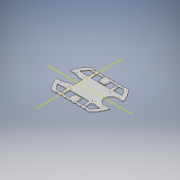
# Autodesk Inventor part: bottomPlate
Saved by Autodesk Inventor 2018 (Build 220112000, 112)
## iProperties
Created: 2020-01-08
Part Number: bottomPlate
Material: Generic
Document SubType Name: Modeling
Designer: anirudh
Density: 1 g/cm^3
Appearance: Default
Author: anirudh
Autodesk Inventor part; units mm, degrees
ref_plane "YZ Plane" through (0, 0, 0) normal (1, 0, 0) x (0, 1, 0)
ref_plane "XZ Plane" through (0, 0, 0) normal (0, 1, 0) x (-1, 0, 0)
ref_plane "XY Plane" through (0, 0, 0) normal (0, 0, 1) x (1, 0, 0)
sketch "Sketch1" plane through (0, 0, 0) normal (0, 1, 0) x (-1, 0, 0)
  arc A0 (-134.4042, 152.4) -> (-189.4285, 73.533) centre (0, 0) ccw
  arc A1 (-189.4285, -73.533) -> (-134.4042, -152.4) centre (0, 0) ccw
  arc A2 (-134.4042, 152.4) -> (-189.4285, 73.533) centre (0, 0) ccw
  arc A3 (-189.4285, -73.533) -> (-134.4042, -152.4) centre (0, 0) ccw
  arc A4 (214.8285, 73.533) -> (159.8042, 152.4) centre (25.4, 0) ccw
  arc A5 (159.8042, -152.4) -> (214.8285, -73.533) centre (25.4, 0) ccw
  arc A6 (214.8285, 73.533) -> (159.8042, 152.4) centre (25.4, 0) ccw
  arc A7 (159.8042, -152.4) -> (214.8285, -73.533) centre (25.4, 0) ccw
  arc A8 (-152.4, -50.8) -> (-152.4, 50.8) centre (-152.4, 0) ccw
  arc A9 (177.8, 50.8) -> (177.8, -50.8) centre (177.8, 0) ccw
  line L0 (177.8, 50.8) -> (222.1476, 50.8)
  line L1 (177.8, -50.8) -> (222.1476, -50.8)
  line L2 (-152.4, 50.8) -> (-196.7476, 50.8)
  line L3 (-152.4, -50.8) -> (-196.7476, -50.8)
  arc A10 (-134.4042, 152.4) -> (-196.7476, 50.8) centre (0, 0) ccw
  arc A11 (-196.7476, -50.8) -> (-134.4042, -152.4) centre (0, 0) ccw
  arc A12 (159.8042, -152.4) -> (222.1476, -50.8) centre (25.4, 0) ccw
  arc A13 (222.1476, 50.8) -> (159.8042, 152.4) centre (25.4, 0) ccw
  circle A14 centre (98.425, -65.0875) radius 2.1
  circle A15 centre (98.425, 65.0875) radius 2.1
  circle A16 centre (-73.025, 65.0875) radius 2.1
  circle A17 centre (-73.025, -65.0875) radius 2.1
  line L4 (-20.32, 152.4) -> (-20.32, 147.32)
  line L5 (-20.32, 147.32) -> (-30.48, 147.32)
  line L6 (-30.48, 147.32) -> (-30.48, 152.4)
  line L7 (-92.5481, 152.4) -> (-92.5481, 147.32)
  line L8 (-92.5481, 147.32) -> (-102.7081, 147.32)
  line L9 (-102.7081, 147.32) -> (-102.7081, 152.4)
  line L10 (-102.7081, 152.4) -> (-134.4042, 152.4)
  line L11 (-60.8521, 152.4) -> (-92.5481, 152.4)
  line L12 (-102.7081, 152.4) -> (-134.4042, 152.4)
  line L13 (-134.4042, 152.4) -> (-102.7081, 152.4)
  line L14 (12.7, 152.4) -> (-20.32, 152.4)
  line L15 (-30.48, 152.4) -> (-60.8521, 152.4)
  line L16 (12.7, 152.4) -> (-20.32, 152.4)
  line L17 (-30.48, 152.4) -> (-92.5481, 152.4)
  line L18 (-92.5481, 152.4) -> (-30.48, 152.4)
  line L19 (-20.32, 152.4) -> (12.7, 152.4)
  line L20 (45.72, 152.4) -> (45.72, 147.32)
  line L21 (45.72, 147.32) -> (55.88, 147.32)
  line L22 (55.88, 147.32) -> (55.88, 152.4)
  line L23 (117.9481, 152.4) -> (117.9481, 147.32)
  line L24 (117.9481, 147.32) -> (128.1081, 147.32)
  line L25 (128.1081, 147.32) -> (128.1081, 152.4)
  line L26 (-20.32, -152.4) -> (-20.32, -147.32)
  line L27 (-20.32, -147.32) -> (-30.48, -147.32)
  line L28 (-30.48, -147.32) -> (-30.48, -152.4)
  line L29 (-92.5481, -152.4) -> (-92.5481, -147.32)
  line L30 (-92.5481, -147.32) -> (-102.7081, -147.32)
  line L31 (-102.7081, -147.32) -> (-102.7081, -152.4)
  line L32 (55.88, -147.32) -> (55.88, -152.4)
  line L33 (45.72, -147.32) -> (55.88, -147.32)
  line L34 (45.72, -152.4) -> (45.72, -147.32)
  line L35 (117.9481, -147.32) -> (128.1081, -147.32)
  line L36 (128.1081, -147.32) -> (128.1081, -152.4)
  line L37 (117.9481, -152.4) -> (117.9481, -147.32)
  line L38 (128.1081, 152.4) -> (159.8042, 152.4)
  line L39 (12.7, 152.4) -> (45.72, 152.4)
  line L40 (55.88, 152.4) -> (117.9481, 152.4)
  line L41 (-102.7081, -152.4) -> (-134.4042, -152.4)
  line L42 (12.7, -152.4) -> (-20.32, -152.4)
  line L43 (-30.48, -152.4) -> (-92.5481, -152.4)
  line L44 (12.7, -152.4) -> (45.72, -152.4)
  line L45 (55.88, -152.4) -> (117.9481, -152.4)
  line L46 (128.1081, -152.4) -> (159.8042, -152.4)
  point P0 (-25.4, -152.4)
  point P1 (50.8, 152.4)
  point P2 (50.8, -152.4)
  point P3 (50.8, -152.4)
  dimension "d22" = 101.6
  dimension "d31" = 4.2
  dimension "d32" = 4.2
  dimension "d34" = 4.2
  constraints: 94 end point, 28 point on circle, 18 centre point, 15 collinear, 12 point on line, 7 perpendicular, 4 coincident, 2 tangent, 1 vertical
  measures "d22" diameter of A9
  measures "d31" diameter of A14
  measures "d32" diameter of A15
  measures "d34" diameter of A17
extrude "Extrusion2" add sketch "Sketch1" along normal blind 5.08
sketch "Sketch2" plane through (0, 5.08, 0) normal (0, 1, 0) x (1, 0, 0)
  arc A0 (-177.8, -50.8) -> (-177.8, 50.8) centre (-177.8, 0) ccw projected
  arc A1 (152.4, 50.8) -> (152.4, -50.8) centre (152.4, 0) ccw projected
  line L0 (-177.8, 0) -> (152.4, 0)
  line L1 (-12.7, 0) -> (-12.7, -152.4)
  line L2 (-12.7, 0) -> (-12.7, 152.4)
  line L3 (20.32, 152.4) -> (-45.72, 152.4) projected
  point P0 (0, 0)
  constraints: 6 end point, 2 midpoint, 1 horizontal
sketch "Sketch3" plane through (0, 5.08, 0) normal (0, 1, 0) x (1, 0, 0)
  circle A0 centre (9.525, 140.4366) radius 1.75
  circle A1 centre (-34.925, 140.4366) radius 1.75
  circle A2 centre (9.525, 102.362) radius 1.75
  circle A3 centre (-34.925, 102.362) radius 1.75
  arc A4 (152.4, 50.8) -> (152.4, -50.8) centre (152.4, 0) ccw projected
  circle A5 centre (9.525, -140.4366) radius 1.75
  circle A6 centre (-34.925, -140.4366) radius 1.75
  circle A7 centre (9.525, -102.362) radius 1.75
  circle A8 centre (-34.925, -102.362) radius 1.75
  point P0 (0, 0)
  dimension "d56" = 3.5
  dimension "d57" = 3.5
  dimension "d58" = 3.5
  constraints: 8 centre point
  measures "d56" diameter of A1
  measures "d57" diameter of A2
  measures "d58" diameter of A3
extrude "Extrusion3" cut sketch "Sketch3" against normal blind 25.4
sketch "Sketch4" plane through (0, 5.08, 0) normal (0, 1, 0) x (1, 0, 0)
  circle A0 centre (-12.7, 0) radius 300
  point P0 (-177.8, 0)
  point P1 (152.4, 0)
  constraints: 1 centre point
sketch "Sketch5" plane through (0, 5.08, 0) normal (0, 1, 0) x (1, 0, 0)
  line L0 (101.6, 0) -> (80.9498, 0)
  arc A0 (-177.8, -50.8) -> (-177.8, 50.8) centre (-177.8, 0) ccw projected
  line L1 (-106.3498, 0) -> (-106.3498, -74.5998)
  line L2 (30.48, -152.4) -> (92.5481, -152.4) projected
  line L3 (80.9498, -74.5998) -> (-106.3498, -74.5998)
  line L4 (-55.88, 152.4) -> (-117.9481, 152.4) projected
  line L5 (-106.3498, 74.5998) -> (80.9498, 74.5998)
  circle A1 centre (9.525, -102.362) radius 1.75 projected
  line L6 (20.32, 152.4) -> (-45.72, 152.4) projected
  circle A2 centre (-34.925, -140.4366) radius 1.75 projected
  line L7 (-41.3004, -140.4366) -> (-41.3004, -152.4)
  line L8 (-45.72, -152.4) -> (20.32, -152.4) projected
  circle A3 centre (-34.925, -102.362) radius 1.75 projected
  line L9 (-34.925, -89.6366) -> (-41.3004, -89.6366)
  line L10 (-41.3004, -89.6366) -> (15.9004, -89.6366)
  circle A4 centre (-34.925, 102.362) radius 1.75 projected
  line L11 (-34.925, 89.6366) -> (-41.3004, 89.6366)
  line L12 (-41.3004, 89.6366) -> (15.9004, 89.6366)
  line L13 (-41.3004, -152.4) -> (-41.3004, -89.6366)
  line L14 (-41.3004, 89.6366) -> (-41.3004, 152.4)
  line L15 (15.9004, -152.4) -> (15.9004, -89.6366)
  line L16 (15.9004, 89.6366) -> (15.9004, 152.4)
  line L17 (80.9498, -74.5998) -> (80.9498, 74.5998)
  line L18 (80.9498, 0) -> (80.9498, -74.5998)
  line L19 (-106.3498, -74.5998) -> (-106.3498, 74.5998)
  arc A5 (134.4042, -152.4) -> (196.7476, -50.8) centre (0, 0) ccw projected
  line L20 (102.7081, -152.4) -> (134.4042, -152.4) projected
  line L21 (80.9498, -74.5998) -> (80.9498, -68.2498)
  line L22 (84.1248, -68.2498) -> (119.6848, -68.2498)
  line L23 (119.6848, -68.2498) -> (119.6848, -86.0298)
  line L24 (119.6848, -86.0298) -> (84.1248, -86.0298)
  line L25 (84.1248, -86.0298) -> (84.1248, -68.2498)
  line L26 (152.4, 0) -> (-177.8, 0)
  line L27 (-12.7, 0) -> (-12.7, 50.8)
  line L28 (-109.5248, -68.2498) -> (-145.0848, -68.2498)
  line L29 (-145.0848, -68.2498) -> (-145.0848, -86.0298)
  line L30 (-145.0848, -86.0298) -> (-109.5248, -86.0298)
  line L31 (-109.5248, -86.0298) -> (-109.5248, -68.2498)
  line L32 (84.1248, 68.2498) -> (119.6848, 68.2498)
  line L33 (119.6848, 68.2498) -> (119.6848, 86.0298)
  line L34 (119.6848, 86.0298) -> (84.1248, 86.0298)
  line L35 (84.1248, 86.0298) -> (84.1248, 68.2498)
  line L36 (-109.5248, 86.0298) -> (-109.5248, 68.2498)
  line L37 (-145.0848, 86.0298) -> (-109.5248, 86.0298)
  line L38 (-145.0848, 68.2498) -> (-145.0848, 86.0298)
  line L39 (-109.5248, 68.2498) -> (-145.0848, 68.2498)
  line L40 (15.9004, -152.4) -> (15.9004, -133.35)
  line L41 (80.9498, -74.5998) -> (63.1698, -74.5998)
  line L42 (63.1698, -82.1182) -> (63.1698, -133.35)
  line L43 (63.1698, -133.35) -> (15.9004, -133.35)
  line L44 (0, -82.1182) -> (63.1698, -82.1182)
  line L45 (84.1248, -133.35) -> (117.6036, -133.35)
  line L46 (84.1248, -133.35) -> (84.1248, -86.0298)
  line L47 (84.1248, -86.0298) -> (155.6011, -86.0298)
  arc A6 (134.4042, -152.4) -> (196.7476, -50.8) centre (0, 0) ccw projected
  arc A7 (117.6036, -133.35) -> (155.6011, -86.0298) centre (0, 0) ccw
  line L48 (63.1698, 82.1182) -> (63.1698, 133.35)
  line L49 (63.1698, 133.35) -> (15.9004, 133.35)
  line L50 (0, 82.1182) -> (63.1698, 82.1182)
  line L51 (84.1248, 133.35) -> (117.6036, 133.35)
  line L52 (84.1248, 133.35) -> (84.1248, 86.0298)
  line L53 (84.1248, 86.0298) -> (155.6011, 86.0298)
  arc A8 (155.6011, 86.0298) -> (117.6036, 133.35) centre (0, 0) ccw
  line L54 (-88.5698, -82.1182) -> (-88.5698, -133.35)
  line L55 (-88.5698, -133.35) -> (-41.3004, -133.35)
  line L56 (-25.4, -82.1182) -> (-88.5698, -82.1182)
  line L57 (-109.5248, -133.35) -> (-143.0036, -133.35)
  line L58 (-109.5248, -133.35) -> (-109.5248, -86.0298)
  line L59 (-109.5248, -86.0298) -> (-181.0011, -86.0298)
  arc A9 (-181.0011, -86.0298) -> (-143.0036, -133.35) centre (-25.4, 0) ccw
  line L60 (-88.5698, 133.35) -> (-41.3004, 133.35)
  line L61 (-88.5698, 82.1182) -> (-88.5698, 133.35)
  line L62 (-25.4, 82.1182) -> (-88.5698, 82.1182)
  line L63 (-109.5248, 133.35) -> (-143.0036, 133.35)
  line L64 (-109.5248, 133.35) -> (-109.5248, 86.0298)
  line L65 (-109.5248, 86.0298) -> (-181.0011, 86.0298)
  arc A10 (-143.0036, 133.35) -> (-181.0011, 86.0298) centre (-25.4, 0) ccw
  line L66 (-41.3004, -133.35) -> (-88.5698, -133.35)
  line L67 (-88.5698, -133.35) -> (-88.5698, -82.1182)
  line L68 (-88.5698, -82.1182) -> (-25.4, -82.1182)
  line L69 (-25.4, -89.6366) -> (-41.3004, -89.6366)
  line L70 (-41.3004, -89.6366) -> (-41.3004, -133.35)
  line L71 (-25.4, -82.1182) -> (0, -82.1182)
  line L72 (-25.4, -89.6366) -> (0, -89.6366)
  line L73 (0, 82.1182) -> (-25.4, 82.1182)
  line L74 (-25.4, 82.1182) -> (-88.5698, 82.1182)
  line L75 (-88.5698, 82.1182) -> (-88.5698, 133.35)
  line L76 (-88.5698, 133.35) -> (-41.3004, 133.35)
  line L77 (-41.3004, 133.35) -> (-41.3004, 89.6366)
  line L78 (-41.3004, 89.6366) -> (-25.4, 89.6366)
  line L79 (15.9004, -133.35) -> (15.9004, -89.6366)
  line L80 (15.9004, -89.6366) -> (-41.3004, -89.6366)
  line L81 (15.9004, 133.35) -> (63.1698, 133.35)
  line L82 (63.1698, 133.35) -> (63.1698, 82.1182)
  line L83 (63.1698, 82.1182) -> (-88.5698, 82.1182)
  line L84 (-88.5698, 82.1182) -> (-88.5698, 133.35)
  line L85 (-88.5698, 133.35) -> (-41.3004, 133.35)
  line L86 (-41.3004, 133.35) -> (-41.3004, 89.6366)
  line L87 (-41.3004, 89.6366) -> (15.9004, 89.6366)
  line L88 (15.9004, 89.6366) -> (15.9004, 133.35)
  constraints: 168 end point, 35 symmetric about line, 20 perpendicular, 9 point on line, 8 collinear, 8 point on circle, 7 horizontal, 4 centre point, 4 parallel, 1 midpoint, 1 vertical, 3 other
ref_plane "Work Plane1" through (134.4042, 0, 0) normal (0, 0, -1) x (-1, 0, 0)
sketch "Sketch6" plane through (0, 5.08, 0) normal (0, 1, 0) x (1, 0, 0)
  arc A0 (196.7476, 50.8) -> (134.4042, 152.4) centre (0, 0) ccw projected
  arc A1 (152.4, 50.8) -> (152.4, -50.8) centre (152.4, 0) ccw projected
  arc A2 (-177.8, -50.8) -> (-177.8, 50.8) centre (-177.8, 0) ccw projected
  line L0 (-45.72, -152.4) -> (20.32, -152.4) projected
  line L1 (20.32, 152.4) -> (-45.72, 152.4) projected
  circle A3 centre (93.0022, 80.3402) radius 1.75
  circle A4 centre (110.7822, 80.3402) radius 1.75
  line L2 (152.4, 0) -> (-177.8, 0)
  line L3 (-12.7, -152.4) -> (-12.7, 152.4)
  circle A5 centre (93.0022, -80.3402) radius 1.75
  circle A6 centre (110.7822, -80.3402) radius 1.75
  circle A7 centre (-118.4022, 80.3402) radius 1.75
  circle A8 centre (-136.1822, 80.3402) radius 1.75
  circle A9 centre (-118.4022, -80.3402) radius 1.75
  circle A10 centre (-136.1822, -80.3402) radius 1.75
  dimension "d86" = 3.5
  dimension "d87" = 3.5
  constraints: 8 centre point, 6 symmetric about line, 4 end point, 2 midpoint, 1 horizontal, 6 other
  measures "d86" diameter of A3
  measures "d87" diameter of A4
extrude "Extrusion4" cut sketch "Sketch6" against normal blind 25.4
extrude "Extrusion5" cut sketch "Sketch5" against normal blind 25.4 contours L49 L48 L50 L73 L62 L61 L60 L14 L11 L12 L16 | L55 L54 L56 L71 L44 L42 L43 L15 L10 L9 L13 | L24 L47 A7 L45 L46 | L58 L57 A9 L59 L30 | L52 L51 A8 L53 L34 | L37 L65 A10 L63 L64
fillet "Fillet1" radius 3.048 4 edges at (15.9004, 2.54, 89.6366) (-41.3004, 2.54, 89.6366) (15.9004, 2.54, -89.6366) (-41.3004, 2.54, -89.6366)
fillet "Fillet2" radius 3.175 28 edges at (63.1698, 2.54, 133.35) (15.9004, 2.54, 133.35) (63.1698, 2.54, 82.1182) (-41.3004, 2.54, 133.35) (-88.5698, 2.54, 133.35) (-88.5698, 2.54, 82.1182) (63.1698, 2.54, -82.1182) (63.1698, 2.54, -133.35) (15.9004, 2.54, -133.35) (-41.3004, 2.54, -133.35) (-88.5698, 2.54, -82.1182) (-88.5698, 2.54, -133.35) (155.6011, 2.54, 86.0298) (84.1248, 2.54, 133.35) (84.1248, 2.54, 86.0298) (117.6036, 2.54, 133.35) (155.6011, 2.54, -86.0298) (117.6036, 2.54, -133.35) (84.1248, 2.54, -133.35) (84.1248, 2.54, -86.0298) (-109.5248, 2.54, 86.0298) (-109.5248, 2.54, 133.35) (-143.0036, 2.54, 133.35) (-181.0011, 2.54, 86.0298) (-109.5248, 2.54, -86.0298) (-109.5248, 2.54, -133.35) (-143.0036, 2.54, -133.35) (-181.0011, 2.54, -86.0298)
fillet "Fillet3" radius 3.175 4 edges at (196.7476, 2.54, 50.8) (196.7476, 2.54, -50.8) (-222.1476, 2.54, 50.8) (-222.1476, 2.54, -50.8)
sketch "Sketch7" plane through (0, 5.08, 0) normal (0, 1, 0) x (1, 0, 0)
  arc A0 (152.4, 50.8) -> (152.4, -50.8) centre (152.4, 0) ccw projected
  circle A1 centre (152.4, -63.5) radius 1.75
  circle A2 centre (152.4, 63.5) radius 1.75
  arc A3 (-177.8, -50.8) -> (-177.8, 50.8) centre (-177.8, 0) ccw projected
  line L0 (152.4, 0) -> (-177.8, 0)
  circle A4 centre (-177.8, -63.5) radius 1.75
  circle A5 centre (-177.8, 63.5) radius 1.75
  dimension "d101" = 3.5
  dimension "d102" = 3.5
  constraints: 4 centre point, 2 end point, 1 horizontal
  measures "d101" diameter of A1
  measures "d102" diameter of A2
extrude "Extrusion6" cut sketch "Sketch7" against normal blind 25.4
sketch "Sketch8" plane through (0, 5.08, 0) normal (0, 1, 0) x (1, 0, 0)
  line L0 (-159.8042, -152.4) -> (-128.1081, -152.4) projected
  line L1 (-159.8042, -152.4) -> (-128.1081, -152.4)
  line L2 (-128.1081, -147.32) -> (-117.9481, -147.32) projected
  line L3 (-128.1081, -152.4) -> (-128.1081, -147.32)
  line L4 (-117.9481, -147.32) -> (-117.9481, -152.4) projected
  line L5 (-128.1081, -147.32) -> (-117.9481, -147.32)
  line L6 (-117.9481, -152.4) -> (-55.88, -152.4) projected
  line L7 (-117.9481, -147.32) -> (-117.9481, -152.4)
  line L8 (-117.9481, -152.4) -> (-55.88, -152.4)
  line L9 (-55.88, -147.32) -> (-45.72, -147.32) projected
  line L10 (-55.88, -152.4) -> (-55.88, -147.32)
  line L11 (-45.72, -147.32) -> (-45.72, -152.4) projected
  line L12 (-55.88, -147.32) -> (-45.72, -147.32)
  line L13 (-45.72, -152.4) -> (20.32, -152.4) projected
  line L14 (-45.72, -147.32) -> (-45.72, -152.4)
  line L15 (-45.72, -152.4) -> (20.32, -152.4)
  line L16 (20.32, -147.32) -> (30.48, -147.32) projected
  line L17 (20.32, -152.4) -> (20.32, -147.32)
  line L18 (30.48, -147.32) -> (30.48, -152.4) projected
  line L19 (20.32, -147.32) -> (30.48, -147.32)
  line L20 (30.48, -147.32) -> (30.48, -152.4)
  line L21 (30.48, -152.4) -> (92.5481, -152.4) projected
  line L22 (30.48, -152.4) -> (92.5481, -152.4)
  line L23 (92.5481, -147.32) -> (102.7081, -147.32) projected
  line L24 (92.5481, -152.4) -> (92.5481, -147.32)
  line L25 (102.7081, -147.32) -> (102.7081, -152.4) projected
  line L26 (92.5481, -147.32) -> (102.7081, -147.32)
  line L27 (102.7081, -147.32) -> (102.7081, -152.4)
  arc A0 (134.4042, -152.4) -> (195.6623, -54.8317) centre (0, 0) ccw projected
  line L28 (102.7081, -152.4) -> (134.4042, -152.4)
  arc A1 (-221.0623, -54.8317) -> (-159.8042, -152.4) centre (-25.4, 0) ccw projected
  line L29 (134.4042, 152.4) -> (102.7081, 152.4) projected
  line L30 (134.4042, 152.4) -> (102.7081, 152.4)
  line L31 (-128.1081, 152.4) -> (-159.8042, 152.4) projected
  line L32 (-128.1081, 147.32) -> (-128.1081, 152.4) projected
  line L33 (-159.8042, 152.4) -> (-128.1081, 152.4)
  line L34 (-117.9481, 147.32) -> (-128.1081, 147.32) projected
  line L35 (-128.1081, 152.4) -> (-128.1081, 147.32)
  line L36 (-128.1081, 147.32) -> (-117.9481, 147.32)
  line L37 (-55.88, 152.4) -> (-117.9481, 152.4) projected
  line L38 (-117.9481, 147.32) -> (-117.9481, 152.4)
  line L39 (-55.88, 147.32) -> (-55.88, 152.4) projected
  line L40 (-117.9481, 152.4) -> (-55.88, 152.4)
  line L41 (-45.72, 147.32) -> (-55.88, 147.32) projected
  line L42 (-55.88, 152.4) -> (-55.88, 147.32)
  line L43 (-55.88, 147.32) -> (-45.72, 147.32)
  line L44 (20.32, 152.4) -> (-45.72, 152.4) projected
  line L45 (-45.72, 147.32) -> (-45.72, 152.4)
  line L46 (-45.72, 152.4) -> (20.32, 152.4)
  line L47 (30.48, 147.32) -> (20.32, 147.32) projected
  line L48 (20.32, 152.4) -> (20.32, 147.32)
  line L49 (20.32, 147.32) -> (30.48, 147.32)
  line L50 (30.48, 152.4) -> (30.48, 147.32) projected
  line L51 (30.48, 147.32) -> (30.48, 152.4)
  line L52 (92.5481, 147.32) -> (92.5481, 152.4) projected
  line L53 (30.48, 152.4) -> (92.5481, 152.4)
  line L54 (92.5481, 152.4) -> (92.5481, 147.32)
  line L55 (102.7081, 152.4) -> (102.7081, 147.32) projected
  line L56 (92.5481, 147.32) -> (102.7081, 147.32)
  line L57 (102.7081, 147.32) -> (102.7081, 152.4)
  arc A2 (-177.8, -50.8) -> (-177.8, 50.8) centre (-177.8, 0) ccw projected
  arc A3 (-177.8, -50.8) -> (-177.8, 50.8) centre (-177.8, 0) ccw
  arc A4 (152.4, 50.8) -> (152.4, -50.8) centre (152.4, 0) ccw projected
  arc A5 (152.4, 50.8) -> (152.4, -50.8) centre (152.4, 0) ccw
  line L58 (152.4, -50.8) -> (196.7476, -50.8)
  line L59 (152.4, 50.8) -> (196.7476, 50.8)
  line L60 (-177.8, -50.8) -> (-218.005, -50.8) projected
  line L61 (-177.8, -50.8) -> (-222.1476, -50.8)
  line L62 (-218.005, 50.8) -> (-177.8, 50.8) projected
  line L63 (-177.8, 50.8) -> (-222.1476, 50.8)
  arc A6 (-159.8042, 152.4) -> (-222.1476, 50.8) centre (-25.4, 0) ccw
  arc A7 (-222.1476, -50.8) -> (-159.8042, -152.4) centre (-25.4, 0) ccw
  arc A8 (134.4042, -152.4) -> (196.7476, -50.8) centre (0, 0) ccw
  arc A9 (196.7476, 50.8) -> (134.4042, 152.4) centre (0, 0) ccw
  line L64 (-177.8, 0) -> (152.4, 0)
  line L65 (-12.7, -80.645) -> (-93.345, -80.645)
  line L66 (-93.345, -80.645) -> (67.945, -80.645)
  line L67 (67.945, -80.645) -> (67.945, 80.645)
  line L68 (67.945, 80.645) -> (-93.345, 80.645)
  line L69 (-93.345, 80.645) -> (-93.345, -80.645)
  circle A10 centre (-177.8, -63.5) radius 1.75 projected
  circle A11 centre (-177.8, -63.5) radius 1.75
  circle A12 centre (-177.8, 63.5) radius 1.75 projected
  circle A13 centre (-177.8, 63.5) radius 1.75
  circle A14 centre (-136.1822, -80.3402) radius 1.75 projected
  circle A15 centre (-136.1822, -80.3402) radius 1.75
  circle A16 centre (-118.4022, -80.3402) radius 1.75 projected
  circle A17 centre (-118.4022, -80.3402) radius 1.75
  circle A18 centre (-136.1822, 80.3402) radius 1.75 projected
  circle A19 centre (-136.1822, 80.3402) radius 1.75
  circle A20 centre (-118.4022, 80.3402) radius 1.75 projected
  circle A21 centre (-118.4022, 80.3402) radius 1.75
  circle A22 centre (93.0022, -80.3402) radius 1.75 projected
  circle A23 centre (93.0022, -80.3402) radius 1.75
  circle A24 centre (110.7822, -80.3402) radius 1.75 projected
  circle A25 centre (110.7822, -80.3402) radius 1.75
  circle A26 centre (152.4, -63.5) radius 1.75 projected
  circle A27 centre (152.4, -63.5) radius 1.75
  circle A28 centre (152.4, 63.5) radius 1.75 projected
  circle A29 centre (152.4, 63.5) radius 1.75
  circle A30 centre (93.0022, 80.3402) radius 1.75 projected
  circle A31 centre (93.0022, 80.3402) radius 1.75
  circle A32 centre (110.7822, 80.3402) radius 1.75 projected
  circle A33 centre (110.7822, 80.3402) radius 1.75
  dimension "d106" = 80.645
  dimension "d107" = 161.29
  constraints: 89 end point, 30 perpendicular, 18 centre point, 16 coincident, 14 point on circle, 7 horizontal, 4 collinear, 4 point on line, 2 parallel, 2 tangent
  measures "d106" distance of L65.start L65.end
  measures "d107" distance of L68.end L67.end
sketch "Sketch10" plane through (0, 5.08, 0) normal (0, 1, 0) x (1, 0, 0)
  line L0 (-177.8, -50.8) -> (-218.005, -50.8) projected
  circle A0 centre (-177.8, -63.5) radius 1.75 projected
  arc A1 (-221.0623, -54.8317) -> (-159.8042, -152.4) centre (-25.4, 0) ccw projected
  circle A2 centre (-209.7483, -57.15) radius 1.75
  circle A3 centre (-188.4494, -57.15) radius 1.75
  line L1 (-218.005, 50.8) -> (-177.8, 50.8) projected
  arc A4 (-177.8, -50.8) -> (-177.8, 50.8) centre (-177.8, 0) ccw projected
  circle A5 centre (-177.8, 63.5) radius 1.75 projected
  arc A6 (-159.8042, 152.4) -> (-221.0623, 54.8317) centre (-25.4, 0) ccw projected
  circle A7 centre (-209.7483, 57.15) radius 1.75
  circle A8 centre (-188.4494, 57.15) radius 1.75
  point P0 (0, 0)
  dimension "d109" = 3.5
  dimension "d110" = 3.5
  dimension "d111" = 3.5
  dimension "d112" = 3.5
  constraints: 4 centre point
  measures "d109" diameter of A2
  measures "d110" diameter of A3
  measures "d111" diameter of A7
  measures "d112" diameter of A8
extrude "Extrusion7" cut sketch "Sketch10" against normal blind 25.4 contours A2 | A3 | A7 | A8
sketch "Sketch12" plane through (0, 5.08, 0) normal (0, 1, 0) x (1, 0, 0)
  arc A0 (-177.8, -50.8) -> (-177.8, 50.8) centre (-177.8, 0) ccw projected
  line L0 (-127, 0) -> (-106.6679, 0)
  circle A1 centre (-116.8339, 0) radius 1.75
  circle A2 centre (-116.8339, 57.15) radius 1.75
  circle A3 centre (-116.8339, -57.15) radius 1.75
  arc A4 (152.4, 50.8) -> (152.4, -50.8) centre (152.4, 0) ccw projected
  circle A5 centre (91.44, 57.15) radius 1.75
  circle A6 centre (91.44, 0) radius 1.75
  circle A7 centre (91.44, -57.15) radius 1.75
  point P0 (0, 0)
  dimension "d120" = 3.5
  dimension "d123" = 3.5
  dimension "d124" = 3.5
  dimension "d128" = 3.5
  dimension "d129" = 3.5
  dimension "d130" = 3.5
  constraints: 6 centre point, 2 end point, 1 horizontal, 1 point on circle
  measures "d120" diameter of A1
  measures "d123" diameter of A2
  measures "d124" diameter of A3
  measures "d128" diameter of A5
  measures "d129" diameter of A6
  measures "d130" diameter of A7
extrude "Extrusion8" cut sketch "Sketch12" against normal blind 25.4
sketch "Sketch13" plane through (0, 5.08, 0) normal (0, 1, 0) x (1, 0, 0)
  line L0 (-107.95, 0) -> (-107.95, 25.4)
  line L1 (-107.95, -25.4) -> (-107.95, 0)
  line L2 (-107.95, -25.4) -> (-107.95, 25.4)
  line L3 (-142.9729, 38.1) -> (-107.95, 38.1)
  line L4 (-107.95, 38.1) -> (-107.95, 25.4)
  line L5 (-142.9729, -38.1) -> (-107.95, -38.1)
  line L6 (-107.95, -38.1) -> (-107.95, -25.4)
  line L7 (-107.95, 38.1) -> (-142.9729, 38.1)
  line L8 (-142.9729, -38.1) -> (-107.95, -38.1)
  line L9 (-107.95, -38.1) -> (-107.95, 38.1)
  line L10 (-107.95, 38.1) -> (-165.6605, 38.1)
  line L11 (-165.6605, 38.1) -> (-165.6605, -38.1)
  line L12 (-165.6605, -38.1) -> (-107.95, -38.1)
  line L13 (-107.95, -38.1) -> (-107.95, 38.1)
  point P0 (0, 0)
  constraints: 28 end point, 3 parallel, 2 horizontal, 1 perpendicular
extrude "Extrusion12" cut sketch "Sketch13" against normal blind 25.4
fillet "Fillet6" radius 3.175 4 edges at (-144.199, 2.54, -38.1) (-107.95, 2.54, -38.1) (-107.95, 2.54, 38.1) (-144.199, 2.54, 38.1)
sketch "Sketch14" plane through (0, 5.08, 0) normal (0, 1, 0) x (1, 0, 0)
  line L0 (92.5481, -152.4) -> (92.5481, -147.32) projected
  line L1 (30.48, -147.32) -> (30.48, -152.4) projected
  line L2 (30.48, -152.4) -> (92.5481, -152.4) projected
  line L3 (66.5941, -152.4) -> (66.5941, -147.32)
  line L4 (66.5941, -147.32) -> (56.4341, -147.32)
  line L5 (56.4341, -147.32) -> (56.4341, -152.4)
  line L6 (-7.62, -152.4) -> (-7.62, -147.32)
  line L7 (-7.62, -147.32) -> (-17.78, -147.32)
  line L8 (-17.78, -147.32) -> (-17.78, -152.4)
  line L9 (-117.9481, -147.32) -> (-117.9481, -152.4) projected
  line L10 (-81.8341, -152.4) -> (-81.8341, -147.32)
  line L11 (-81.8341, -147.32) -> (-91.9941, -147.32)
  line L12 (-91.9941, -147.32) -> (-91.9941, -152.4)
  line L13 (66.5941, -152.4) -> (56.4341, -152.4)
  line L14 (-7.62, -152.4) -> (-17.78, -152.4)
  line L15 (-45.72, -152.4) -> (20.32, -152.4) projected
  line L16 (-81.8341, -152.4) -> (-91.9941, -152.4)
  line L17 (-117.9481, -152.4) -> (-55.88, -152.4) projected
  line L18 (-107.95, 34.925) -> (-107.95, -34.925) projected
  line L19 (-107.95, 0) -> (128.2079, 0)
  line L20 (-107.95, 0) -> (167.8207, 0)
  line L21 (92.5481, 152.4) -> (92.5481, 147.32)
  line L22 (66.5941, 152.4) -> (66.5941, 147.32)
  line L23 (66.5941, 147.32) -> (56.4341, 147.32)
  line L24 (56.4341, 147.32) -> (56.4341, 152.4)
  line L25 (-7.62, 152.4) -> (-7.62, 147.32)
  line L26 (-7.62, 147.32) -> (-17.78, 147.32)
  line L27 (-17.78, 147.32) -> (-17.78, 152.4)
  line L28 (-117.9481, 147.32) -> (-117.9481, 152.4)
  line L29 (-81.8341, 152.4) -> (-81.8341, 147.32)
  line L30 (-81.8341, 147.32) -> (-91.9941, 147.32)
  line L31 (-91.9941, 147.32) -> (-91.9941, 152.4)
  line L32 (66.5941, 152.4) -> (56.4341, 152.4)
  line L33 (-7.62, 152.4) -> (-17.78, 152.4)
  line L34 (-81.8341, 152.4) -> (-91.9941, 152.4)
  point P0 (0, 0)
  dimension "d151" = 5.08
  dimension "d152" = 10.16
  dimension "d154" = 5.08
  dimension "d155" = 10.16
  constraints: 56 end point, 16 symmetric about line, 5 perpendicular, 3 collinear, 2 point on line, 1 midpoint
  measures "d151" distance of L3.start L3.end
  measures "d152" distance of L3.end L4.end
  measures "d154" distance of L6.start L6.end
  measures "d155" distance of L6.end L7.end
extrude "Extrusion13" cut sketch "Sketch14" against normal blind 25.4
ref_plane "Work Plane2" through (-99.0473, 5.08, 89.2048) normal (-1, 0, 0) x (0, 0, 1)
sketch "Sketch16" plane through (0, 5.08, 0) normal (0, 1, 0) x (1, 0, 0)
  line L0 (-112.6998, -133.35) -> (-141.7974, -133.35) projected
  line L1 (-112.6998, -133.35) -> (-138.0998, -133.35)
  line L2 (-44.4754, -133.35) -> (-85.3948, -133.35) projected
  line L3 (-85.3948, -133.35) -> (-59.9948, -133.35)
  arc A0 (-112.6998, -133.35) -> (-109.5248, -130.175) centre (-112.6998, -130.175) ccw projected
  arc A1 (-112.6998, -133.35) -> (-109.5248, -130.175) centre (-112.6998, -130.175) ccw
  arc A2 (-88.5698, -130.175) -> (-85.3948, -133.35) centre (-85.3948, -130.175) ccw projected
  arc A3 (-88.5698, -130.175) -> (-85.3948, -133.35) centre (-85.3948, -130.175) ccw
  line L4 (-109.5248, -130.175) -> (-109.5248, -117.475)
  line L5 (-109.5248, -89.2048) -> (-109.5248, -130.175) projected
  line L6 (-109.5248, -117.475) -> (-88.5698, -117.475)
  line L7 (-88.5698, -130.175) -> (-88.5698, -85.2932) projected
  line L8 (-88.5698, -117.475) -> (-88.5698, -130.175)
  line L9 (-128.1081, -147.32) -> (-117.9481, -147.32) projected
  line L10 (-138.0998, -141.732) -> (-138.0998, -133.35)
  line L11 (-59.9948, -141.732) -> (-59.9948, -133.35)
  line L12 (-109.5248, -117.475) -> (-88.5698, -117.475)
  circle A4 centre (-104.2861, -123.825) radius 1.75
  circle A5 centre (-93.8086, -123.825) radius 1.75
  circle A6 centre (-99.0473, -132.4201) radius 1.75
  line L13 (-138.0998, -141.732) -> (-59.9948, -141.732)
  line L14 (-107.95, 34.925) -> (-107.95, -34.925) projected
  arc A7 (152.4, 50.8) -> (152.4, -50.8) centre (152.4, 0) ccw projected
  arc A8 (-177.8, -50.8) -> (-145.0655, -38.8471) centre (-177.8, 0) ccw projected
  line L15 (152.4, 0) -> (-177.8, 0)
  line L16 (-12.7, 0) -> (-12.7, -231.0241)
  line L17 (87.2998, -133.35) -> (116.3974, -133.35)
  line L18 (87.2998, -133.35) -> (112.6998, -133.35)
  line L19 (59.9948, -133.35) -> (34.5948, -133.35)
  arc A9 (84.1248, -130.175) -> (87.2998, -133.35) centre (87.2998, -130.175) ccw
  arc A10 (84.1248, -130.175) -> (87.2998, -133.35) centre (87.2998, -130.175) ccw
  arc A11 (59.9948, -133.35) -> (63.1698, -130.175) centre (59.9948, -130.175) ccw
  arc A12 (59.9948, -133.35) -> (63.1698, -130.175) centre (59.9948, -130.175) ccw
  line L20 (84.1248, -130.175) -> (84.1248, -117.475)
  line L21 (84.1248, -117.475) -> (63.1698, -117.475)
  line L22 (63.1698, -117.475) -> (63.1698, -130.175)
  line L23 (102.7081, -147.32) -> (92.5481, -147.32)
  line L24 (112.6998, -141.732) -> (112.6998, -133.35)
  line L25 (34.5948, -141.732) -> (34.5948, -133.35)
  line L26 (84.1248, -117.475) -> (63.1698, -117.475)
  circle A13 centre (78.8861, -123.825) radius 1.75
  circle A14 centre (68.4086, -123.825) radius 1.75
  circle A15 centre (73.6473, -132.4201) radius 1.75
  line L27 (112.6998, -141.732) -> (34.5948, -141.732)
  line L28 (-112.6998, 133.35) -> (-141.7974, 133.35)
  line L29 (-112.6998, 133.35) -> (-138.0998, 133.35)
  line L30 (-85.3948, 133.35) -> (-59.9948, 133.35)
  arc A16 (-109.5248, 130.175) -> (-112.6998, 133.35) centre (-112.6998, 130.175) ccw
  arc A17 (-109.5248, 130.175) -> (-112.6998, 133.35) centre (-112.6998, 130.175) ccw
  arc A18 (-85.3948, 133.35) -> (-88.5698, 130.175) centre (-85.3948, 130.175) ccw
  arc A19 (-85.3948, 133.35) -> (-88.5698, 130.175) centre (-85.3948, 130.175) ccw
  line L31 (-109.5248, 130.175) -> (-109.5248, 117.475)
  line L32 (-109.5248, 117.475) -> (-88.5698, 117.475)
  line L33 (-88.5698, 117.475) -> (-88.5698, 130.175)
  line L34 (-138.0998, 141.732) -> (-138.0998, 133.35)
  line L35 (-59.9948, 141.732) -> (-59.9948, 133.35)
  line L36 (-109.5248, 117.475) -> (-88.5698, 117.475)
  circle A20 centre (-104.2861, 123.825) radius 1.75
  circle A21 centre (-93.8086, 123.825) radius 1.75
  circle A22 centre (-99.0473, 132.4201) radius 1.75
  line L37 (-138.0998, 141.732) -> (-59.9948, 141.732)
  line L38 (87.2998, 133.35) -> (116.3974, 133.35)
  circle A23 centre (73.6473, 132.4201) radius 1.75
  arc A24 (87.2998, 133.35) -> (84.1248, 130.175) centre (87.2998, 130.175) ccw
  arc A25 (63.1698, 130.175) -> (59.9948, 133.35) centre (59.9948, 130.175) ccw
  arc A26 (87.2998, 133.35) -> (84.1248, 130.175) centre (87.2998, 130.175) ccw
  line L39 (87.2998, 133.35) -> (112.6998, 133.35)
  line L40 (112.6998, 141.732) -> (112.6998, 133.35)
  line L41 (112.6998, 141.732) -> (34.5948, 141.732)
  arc A27 (63.1698, 130.175) -> (59.9948, 133.35) centre (59.9948, 130.175) ccw
  line L42 (59.9948, 133.35) -> (34.5948, 133.35)
  line L43 (34.5948, 141.732) -> (34.5948, 133.35)
  circle A28 centre (68.4086, 123.825) radius 1.75
  circle A29 centre (78.8861, 123.825) radius 1.75
  line L44 (63.1698, 117.475) -> (63.1698, 130.175)
  line L45 (84.1248, 130.175) -> (84.1248, 117.475)
  line L46 (84.1248, 117.475) -> (63.1698, 117.475)
  line L47 (84.1248, 117.475) -> (63.1698, 117.475)
  point P0 (0, 0)
  constraints: 85 end point, 56 symmetric about line, 28 point on circle, 26 centre point, 8 coincident, 7 point on line, 5 perpendicular, 1 collinear, 1 horizontal, 1 midpoint, 1 tangent, 21 other
extrude "Extrusion15" cut sketch "Sketch16" against normal blind 25.4 contours A4 | A5 | A6 | A13 | A14 | A15 | A20 | A21 | A22 | A23 | A28 | A29
body "Solid2"
